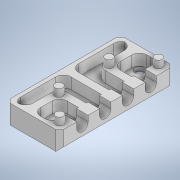
# Autodesk Inventor part: Штекер
Saved by Autodesk Inventor 2020 (Build 240168000, 168)
## iProperties
Created: 2021-06-08
Part Number: Штекер
Material: Типовые
Document SubType Name: Modeling
Designer: I_Love_U_Bogdan
Density: 1 g/cm^3
Appearance: По умолчанию
Author: I_Love_U_Bogdan
Autodesk Inventor part; units mm, degrees
ref_plane "YZ Plane" through (0, 0, 0) normal (1, 0, 0) x (0, 1, 0)
ref_plane "XZ Plane" through (0, 0, 0) normal (0, 1, 0) x (-1, 0, 0)
ref_plane "XY Plane" through (0, 0, 0) normal (0, 0, 1) x (1, 0, 0)
sketch "Эскиз10" plane through (0, 0, 0) normal (0, 1, 0) x (-1, 0, 0)
  line L0 (-2.5, 7.5) -> (2.5, 7.5)
  line L1 (2.5, 7.5) -> (2.5, -7.5)
  line L2 (2.5, -7.5) -> (-2.5, -7.5)
  line L3 (-2.5, -7.5) -> (-2.5, 7.5)
  line L4 (-2.5, 7.5) -> (2.5, -7.5) construction
  line L5 (2.5, 7.5) -> (-2.5, -7.5) construction
  line L6 (2.5, -7.5) -> (0, -7.5)
  line L7 (0, -7.5) -> (0, -5)
  line L8 (0, -5) -> (2.5, -5)
  line L9 (2.5, -5) -> (2.5, -7.5)
  line L10 (2.5, -5) -> (0, -7.5)
  line L11 (0, -5) -> (2.5, -7.5)
  circle A0 centre (1.25, -6.25) radius 0.6
  circle A1 centre (-1.25, -6.25) radius 0.6
  line L12 (2.5, 0) -> (-2.5, 0)
  point P0 (0, 0)
  dimension "d48" = 5
  dimension "d49" = 15
  dimension "d50" = 2.5
  dimension "d51" = 2.5
  dimension "d52" = 1.2
  dimension "d53" = 1.25
  dimension "d54" = 1.25
  dimension "d55" = 1.2
  dimension "d56" = 1.25
  constraints: 26 end point, 5 midpoint, 4 parallel, 3 perpendicular, 2 centre point, 2 horizontal
  measures "d48" distance of L1.end L2.end
  measures "d49" distance of L0.end L1.end
  measures "d50" distance of L7.end L8.end
  measures "d51" distance of L6.end L7.end
  measures "d52" diameter of A0
  measures "d53" distance from line of L3 A1.centre
  measures "d54" distance from line of L2 A1.centre
  measures "d55" diameter of A1
  measures "d56" distance from line of L9 A0.centre
extrude "Выдавливание10" add sketch "Эскиз10" along normal blind 1 contours L12 L1 L8 L7 L2 L3 | L10 A0 L11 L8 | L1 L11 A0 L10 | L10 A0 L11 L2 | L7 L11 A0 L10
sketch "Эскиз12" plane through (0, 0, 0) normal (0, -1, 0) x (1, 0, 0)
  line L0 (2.5, 0) -> (2.5, -7.5) projected
  line L1 (2.5, 0) -> (4.5, 0)
  line L2 (4.5, 0) -> (4.5, -7.5)
  line L3 (4.5, -7.5) -> (2.5, -7.5)
  line L4 (2.5, -7.5) -> (2.5, 0)
  point P0 (0, 0)
  dimension "d65" = 2
  constraints: 8 end point, 2 parallel, 1 horizontal, 1 perpendicular
  measures "d65" distance of L2.end L3.end
extrude "Выдавливание12" add sketch "Эскиз12" against normal blind 1
sketch "Эскиз13" plane through (0, 1, 0) normal (0, 1, 0) x (1, 0, 0)
  line L0 (-2.5, 7.5) -> (-2.5, 0) projected
  line L1 (4.5, 7.5) -> (-2.5, 7.5) projected
  line L2 (-2, 0) -> (-2, 7)
  line L3 (-2, 7) -> (4.5, 7)
  line L4 (-2.5, 0) -> (4.5, 0) projected
  line L5 (4.5, 0) -> (4.5, 7.5) projected
  line L6 (3, 7) -> (3, 0)
  point P0 (0, 0)
  dimension "d68" = 0.5
  dimension "d71" = 1.5
  constraints: 6 end point, 2 point on line, 1 perpendicular, 1 other
  measures "d68" distance between parallel lines of L0 L2
  measures "d71" distance between parallel lines of L5 L6
extrude "Выдавливание13" add sketch "Эскиз13" along normal blind 1.5 contours L1 L5 L3 L2 L4 L0 | L5 L4 L6 L3
sketch "Эскиз14" plane through (4.5, 0, 0) normal (1, 0, 0) x (0, 0, -1)
  line L0 (0, 1) -> (7, 1) projected
  line L1 (7.5, 0) -> (0, 0) projected
  line L2 (7.5, 0) -> (7.5, 2.5) projected
  line L3 (0, 2.5) -> (7.5, 2.5) projected
  line L4 (0, 0) -> (0, 2.5) projected
  circle A0 centre (1.5, 1.75) radius 0.75
  circle A1 centre (4.5, 1.75) radius 0.75
  line L5 (0, 2.5) -> (7.5, 2.5) projected
  line L6 (0.75, 2.5) -> (2.25, 2.5)
  line L7 (2.25, 2.5) -> (2.25, 1.75)
  line L8 (2.25, 1.75) -> (0.75, 1.75)
  line L9 (0.75, 1.75) -> (0.75, 2.5)
  line L10 (3.75, 2.5) -> (5.25, 2.5)
  line L11 (5.25, 2.5) -> (5.25, 1.75)
  line L12 (5.25, 1.75) -> (3.75, 1.75)
  line L13 (3.75, 1.75) -> (3.75, 2.5)
  point P0 (0, 0)
  dimension "d72" = 1.5
  dimension "d73" = 1.5
  dimension "d74" = 3
  dimension "d75" = 3
  dimension "d76" = 0.75
  constraints: 16 end point, 4 parallel, 4 vertical, 2 horizontal, 2 perpendicular, 1 midpoint, 1 point on line, 6 other
  measures "d74" distance from line of L2 point (4.5, 1.75)
  measures "d75" distance of point (4.5, 1.75) point (1.5, 1.75)
  measures "d76" distance from line of L3 point (4.5, 1.75)
extrude "Выдавливание14" cut sketch "Эскиз14" against normal blind 1.5 contours A0 L8 | A1 L12 | L9 L3 A0 | A0 L8 | A0 L3 L7 | L13 L3 A1 | A1 L12 | A1 L3 L11
sketch "Эскиз15" plane through (0, 1, 0) normal (0, 1, 0) x (1, 0, 0)
  circle A0 centre (-1.25, 6.25) radius 0.6 projected
  circle A1 centre (1.25, 6.25) radius 0.6 projected
  circle A2 centre (1.25, 6.25) radius 1.1
  circle A3 centre (-1.25, 6.25) radius 1.1
  line L0 (3, 3.75) -> (3, 2.25) projected
  line L1 (3, 3) -> (0, 3)
  line L2 (0, 3) -> (0, 6.25)
  line L3 (-1.25, 6.25) -> (1.25, 6.25)
  line L4 (3, 3.5) -> (0.5, 3.5)
  line L5 (0.5, 3.5) -> (0.5, 7)
  line L6 (3, 2.5) -> (-0.5, 2.5)
  line L7 (-0.5, 2.5) -> (-0.5, 7)
  line L8 (-2, 0) -> (3, 0) projected
  line L9 (-2, 0.5) -> (3, 0.5)
  line L10 (-2, 7) -> (3, 7) projected
  line L11 (-2, 0) -> (-2, 7) projected
  line L12 (4.5, 0.75) -> (3, 0.75) projected
  line L13 (3, 0.75) -> (3, 0) projected
  line L14 (3, 0) -> (4.5, 0) projected
  line L15 (4.5, 0) -> (4.5, 0.75) projected
  line L16 (3, 0.75) -> (3, 0) projected
  point P0 (0, 0)
  point P1 (3, 0.5)
  dimension "d79" = 0.5
  dimension "d80" = 0.5
  dimension "d81" = 0.5
  dimension "d82" = 0.5
  dimension "d83" = 0.5
  constraints: 16 end point, 3 midpoint, 2 centre point, 2 horizontal, 1 parallel, 1 point on line
  measures "d79" radial gap between concentric circles of A1 A2
  measures "d80" radial gap between concentric circles of A0 A3
  measures "d81" distance between parallel lines of L1 L4
  measures "d82" distance between parallel lines of L1 L6
  measures "d83" distance between parallel lines of L8 L9
extrude "Выдавливание15" add sketch "Эскиз15" along normal blind 1.5 contours L5 L4 L0 L1 L2 L3 A2 | A2 L3 L5 | L10 L5 L3 A2 | A2 L3 A3 L10 | A3 L3 L7 L10 | L2 L1 L0 L6 L7 A3 L3 | A3 L7 L3 | L11 L9 L13 L8
fillet "Сопряжение1" radius 1 7 edges at (-0.5, 1.75, -2.5) (0.5, 1.75, -3.5) (-2, 1.75, -0.5) (0.5, 1.75, -7) (-0.5, 1.75, -7) (-2, 1.75, -7) (3, 1.75, -7)
sketch "Эскиз16" plane through (0, 2.5, 0) normal (0, 1, 0) x (1, 0, 0)
  circle A0 centre (3.5, 6.5) radius 0.5
  line L0 (4.5, 5.25) -> (4.5, 7.5) projected
  line L1 (4.5, 7.5) -> (-2.5, 7.5) projected
  circle A1 centre (0.2, 3.3) radius 0.5
  line L2 (-2.5, 7.5) -> (-2.5, 0) projected
  point P0 (0, 0)
  dimension "d90" = 1
  dimension "d91" = 1
  dimension "d92" = 1
  dimension "d93" = 1
  dimension "d94" = 4.2
  dimension "d95" = 2.7
  constraints: 2 centre point
  measures "d90" diameter of A0
  measures "d91" distance from line of L0 A0.centre
  measures "d92" distance from line of L1 A0.centre
  measures "d93" diameter of A1
  measures "d94" distance from line of L1 A1.centre
  measures "d95" distance from line of L2 A1.centre
extrude "Выдавливание16" add sketch "Эскиз16" along normal blind 1
mirror "Зеркальное отражение1" about plane through (-2.5, 0, 0) normal (0, 0, 1)
chamfer "Фаска2" distance 0.5 angle 45 9 edges at (-0.65, 0, -6.25) (1.85, 0, -6.25) (-0.65, 0, 6.25) (1.85, 0, 6.25) (4.5, 1.25, -7.5) (4.5, 0, 0) (4.5, 1.25, 7.5) (-2.5, 1.25, -7.5) (-2.5, 1.25, 7.5)
sketch "Эскиз18" plane through (0, 18.25, 0) normal (0, 1, 0) x (1, 0, 0)
  line L0 (4.5, -7) -> (4, -7.5) projected
  line L1 (4.5, -5.25) -> (4.5, -7) projected
  line L2 (3, -5.25) -> (4.5, -5.25) projected
  line L3 (3, -6) -> (3, -5.25) projected
  arc A0 (2, -7) -> (3, -6) centre (2, -6) ccw projected
  line L4 (1.5, -7) -> (2, -7) projected
  arc A1 (0.5, -6) -> (1.5, -7) centre (1.5, -6) ccw projected
  line L5 (0.5, -4.5) -> (0.5, -6) projected
  arc A2 (1.5, -3.5) -> (0.5, -4.5) centre (1.5, -4.5) ccw projected
  line L6 (3, -3.5) -> (1.5, -3.5) projected
  line L7 (3, -3.75) -> (3, -3.5) projected
  line L8 (4.5, -3.75) -> (3, -3.75) projected
  line L9 (4.5, -2.25) -> (4.5, -3.75) projected
  line L10 (3, -2.25) -> (4.5, -2.25) projected
  line L11 (3, -2.5) -> (3, -2.25) projected
  line L12 (0.5, -2.5) -> (3, -2.5) projected
  arc A3 (0.5, -2.5) -> (-0.5, -3.5) centre (0.5, -3.5) ccw projected
  line L13 (-0.5, -6) -> (-0.5, -3.5) projected
  arc A4 (-1.5, -7) -> (-0.5, -6) centre (-1.5, -6) ccw projected
  arc A5 (-2, -6.134) -> (-1.5, -7) centre (-1, -6.134) ccw projected
  line L14 (-2, -1.5) -> (-2, -6.134) projected
  arc A6 (-1, -0.5) -> (-2, -1.5) centre (-1, -1.5) ccw projected
  line L15 (3, -0.5) -> (-1, -0.5) projected
  line L16 (3, -0.75) -> (3, -0.5) projected
  line L17 (4.5, -0.75) -> (3, -0.75) projected
  line L18 (4.5, 0.75) -> (4.5, -0.75) projected
  line L19 (4.5, 0.75) -> (3, 0.75) projected
  line L20 (3, 0.75) -> (3, 0.5) projected
  line L21 (3, 0.5) -> (-1, 0.5) projected
  arc A7 (-2, 1.5) -> (-1, 0.5) centre (-1, 1.5) ccw projected
  line L22 (-2, 1.5) -> (-2, 6.134) projected
  arc A8 (-1.5, 7) -> (-2, 6.134) centre (-1, 6.134) ccw projected
  arc A9 (-0.5, 6) -> (-1.5, 7) centre (-1.5, 6) ccw projected
  line L23 (-0.5, 6) -> (-0.5, 3.5) projected
  arc A10 (-0.5, 3.5) -> (0.5, 2.5) centre (0.5, 3.5) ccw projected
  line L24 (0.5, 2.5) -> (3, 2.5) projected
  line L25 (3, 2.5) -> (3, 2.25) projected
  line L26 (3, 2.25) -> (4.5, 2.25) projected
  line L27 (4.5, 2.25) -> (4.5, 3.75) projected
  line L28 (4.5, 3.75) -> (3, 3.75) projected
  line L29 (3, 3.75) -> (3, 3.5) projected
  line L30 (3, 3.5) -> (1.5, 3.5) projected
  arc A11 (0.5, 4.5) -> (1.5, 3.5) centre (1.5, 4.5) ccw projected
  line L31 (0.5, 4.5) -> (0.5, 6) projected
  arc A12 (1.5, 7) -> (0.5, 6) centre (1.5, 6) ccw projected
  line L32 (1.5, 7) -> (2, 7) projected
  arc A13 (3, 6) -> (2, 7) centre (2, 6) ccw projected
  line L33 (3, 6) -> (3, 5.25) projected
  line L34 (3, 5.25) -> (4.5, 5.25) projected
  line L35 (4.5, 5.25) -> (4.5, 7) projected
  line L36 (4, 7.5) -> (4.5, 7) projected
  line L37 (4, 7.5) -> (-2, 7.5) projected
  line L38 (-2.5, 7) -> (-2.5, -7) projected
  line L39 (4, -7.5) -> (-2, -7.5) projected
  circle A14 centre (0.2, -3.3) radius 0.5 projected
  circle A15 centre (3.5, -6.5) radius 0.5 projected
  circle A16 centre (3.5, 6.5) radius 0.5 projected
  circle A17 centre (0.2, 3.3) radius 0.5 projected
  line L40 (-2, -7.5) -> (-2.5, -7) projected
  line L41 (-2.5, 7) -> (-2, 7.5) projected
  line L42 (4.5, -5.25) -> (3, -5.25) projected
  line L43 (4.5, -5.25) -> (4.5, 5.25)
  circle A18 centre (0.2, -3.3) radius 0.6
  circle A19 centre (3.5, -6.5) radius 0.6
  circle A20 centre (0.2, 3.3) radius 0.6
  circle A21 centre (3.5, 6.5) radius 0.6
  point P0 (0, 0)
  dimension "d99" = 0.1
  dimension "d100" = 0.1
  dimension "d101" = 0.1
  dimension "d102" = 0.1
  constraints: 4 centre point, 2 end point, 1 perpendicular
  measures "d99" radial gap between concentric circles of A14 A18
  measures "d100" radial gap between concentric circles of A15 A19
  measures "d101" radial gap between concentric circles of A17 A20
  measures "d102" radial gap between concentric circles of A16 A21
